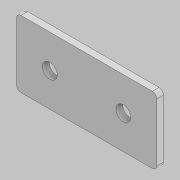
# Autodesk Inventor part: rocker_bogie_mount
Saved by Autodesk Inventor 2021.2 (Build 252289000, 289)
## iProperties
Created: 2021-07-09
Part Number: rocker_bogie_mount
Material: Generic
Document SubType Name: Modeling
Designer: gisen
Density: 1 g/cm^3
Appearance: Default
Author: gisen
Autodesk Inventor part; units mm, degrees
ref_plane "YZ Plane" through (0, 0, 0) normal (1, 0, 0) x (0, 1, 0)
ref_plane "XZ Plane" through (0, 0, 0) normal (0, 1, 0) x (-1, 0, 0)
ref_plane "XY Plane" through (0, 0, 0) normal (0, 0, 1) x (1, 0, 0)
sketch "スケッチ2" plane through (0, 0, 0) normal (0, 0, 1) x (1, 0, 0)
  line L0 (-31.5, 15) -> (31.5, 15)
  line L1 (31.5, 15) -> (31.5, -15)
  line L2 (31.5, -15) -> (-31.5, -15)
  line L3 (-31.5, -15) -> (-31.5, 15)
  line L4 (0, 21) -> (0, -21) construction
  line L5 (-44.1, 0) -> (44.1, 0) construction
  point P0 (0, 0)
  dimension "d1" = 63
  dimension "d2" = 30
  dimension "d3" = 15
  dimension "d4" = 31.5
  constraints: 8 end point, 2 parallel, 1 horizontal, 1 perpendicular
  measures "d1" distance of L1.end L2.end
  measures "d2" distance of L0.end L1.end
  measures "d3" distance between parallel lines of L0 L5
  measures "d4" distance between parallel lines of L4 L3
extrude "押し出し1" add sketch "スケッチ2" along normal blind 3
sketch "スケッチ3" plane through (0, 0, 3) normal (0, 0, 1) x (1, 0, 0)
  line L0 (-31.5, -15) -> (31.5, -15) construction
  line L1 (31.5, -15) -> (31.5, 15) construction
  line L2 (31.5, 15) -> (-31.5, 15) construction
  line L3 (-31.5, 15) -> (-31.5, -15) construction
  line L4 (-44.1, 0) -> (44.1, 0) construction
  point P0 (0, 0)
  point P1 (-16.5, 0)
  point P2 (16.5, 0)
  dimension "d7" = 15
  dimension "d8" = 15
  constraints: 2 point on line
  measures "d7" distance from line of point (-16.5, 0) L3
  measures "d8" distance from line of L1 point (16.5, 0)
hole "穴1" at (-16.5, 0, 3) at (16.5, 0, 3) direction (0, 0, -1) diameter 6.6 end through all
fillet "フィレット1" radius 2 4 edges at (-31.5, 15, 1.5) (31.5, 15, 1.5) (31.5, -15, 1.5) (-31.5, -15, 1.5)
equation "\"d3\" = 0.5 * d2"
equation "\"d4\" = 0.5 * d1"
